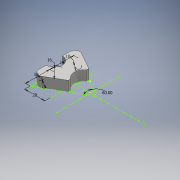
# Autodesk Inventor part: 240412_sketch3
Saved by Autodesk Inventor 2016 (Build 200138000, 138)
## iProperties
Created: 2024-04-12
Part Number: 240412_sketch3
Material: 일반
Document SubType Name: Modeling
Designer: pc
Density: 1 g/cm^3
Appearance: 기본값
Author: pc
Autodesk Inventor part; units mm, degrees
ref_plane "YZ Plane" through (0, 0, 0) normal (1, 0, 0) x (0, 1, 0)
ref_plane "XZ Plane" through (0, 0, 0) normal (0, 1, 0) x (-1, 0, 0)
ref_plane "XY Plane" through (0, 0, 0) normal (0, 0, 1) x (1, 0, 0)
sketch "스케치1" plane through (0, 0, 0) normal (0, 0, 1) x (1, 0, 0)
  line L0 (-0.0808, 29.1134) -> (-0.0808, -34.3055)
  line L1 (-44.0255, 0.0549) -> (53.8558, 0.0549)
  line L2 (-35.8687, -7.9451) -> (-35.8687, -23.9451)
  line L3 (-35.8687, -23.9451) -> (-35.8687, 0.0549)
  line L4 (-35.8687, 8.0549) -> (-35.8687, 24.0549)
  line L5 (-35.8687, 24.0549) -> (5.7005, 0.0549)
  line L6 (-35.8687, -23.9451) -> (5.7005, 0.0549)
  arc A0 (-35.8687, -15.2849) -> (-28.3687, -19.615) centre (-30.8687, -15.2849) ccw
  arc A1 (-28.3687, 19.7248) -> (-35.8687, 15.3946) centre (-30.8687, 15.3946) ccw
  arc A2 (-35.8687, -7.9451) -> (-35.8687, 8.0549) centre (-35.8687, 0.0549) ccw
  line L7 (-15.8687, 16.9552) -> (-15.8687, -23.9451)
  arc A3 (-11.8687, 8.0549) -> (-11.8687, -7.9451) centre (-5.8687, 0.0549) ccw
  line L8 (-11.8687, 10.1985) -> (-11.8687, 8.0549)
  line L9 (-11.8687, -7.9451) -> (-11.8687, -10.0887)
  dimension "d7" = 24
  dimension "d8" = 24
  dimension "d9" = 60
  dimension "d10" = 10
  dimension "d11" = 10
  dimension "d12" = 16
  dimension "d14" = 20
  constraints: 20 end point, 10 point on line, 8 point on circle, 5 tangent, 5 vertical, 4 centre point, 1 coincident, 1 horizontal, 1 parallel, 1 perpendicular
  measures "d7" distance of L3.end L2.end
  measures "d8" distance of L3.end L4.end
  measures "d9" angle of L6 L5
  measures "d10" diameter of A0
  measures "d11" diameter of A1
  measures "d12" diameter of A2
  measures "d14" distance between parallel lines of L2 L7
sketch "스케치2" plane through (0, 0, 0) normal (0, 0, 1) x (1, 0, 0)
  point P0 (0, 0)
extrude "돌출1" add sketch "스케치1" along normal blind 10 contours L8 A3 L7 L5 | L7 L6 A0 L2 A2 L1 | L1 A2 L4 A1 L5 L7 | A3 L9 L6 L7
sketch "스케치3" plane through (0, 0, 10) normal (0, 0, 1) x (1, 0, 0)
  point P0 (0, 0)
sketch "스케치4" plane through (0, 0, 10) normal (0, 0, 1) x (1, 0, 0)
  point P0 (0, 0)
